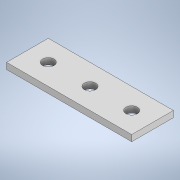
# Autodesk Inventor part: X-Axis End Pulley Holder
Saved by Autodesk Inventor 2022 (Build 260153000, 153)
## iProperties
Created: 2022-12-29
Part Number: X-Axis End Pulley Holder
Material: Generic
Document SubType Name: Modeling
Designer: Gaming
Density: 1 g/cm^3
Appearance: Default
Author: Gaming
Autodesk Inventor part; units mm, degrees
ref_plane "YZ Plane" through (0, 0, 0) normal (1, 0, 0) x (0, 1, 0)
ref_plane "XZ Plane" through (0, 0, 0) normal (0, 1, 0) x (-1, 0, 0)
ref_plane "XY Plane" through (0, 0, 0) normal (0, 0, 1) x (1, 0, 0)
sketch "Sketch1" plane through (0, 0, 0) normal (0, 1, 0) x (-1, 0, 0)
  line L0 (30, 10) -> (-30, 10)
  line L1 (-30, 10) -> (-30, -10)
  line L2 (-30, -10) -> (30, -10)
  line L3 (30, -10) -> (30, 10)
  point P0 (0, 0)
  point P1 (30, 0)
  point P2 (0, -10)
  dimension "d0" = 60
  dimension "d1" = 20
  constraints: 8 end point, 2 midpoint, 2 parallel, 1 horizontal, 1 horizontal alignment, 1 perpendicular, 1 vertical alignment
  measures "d0" distance of L2.end L1.end
  measures "d1" distance of L1.end L0.end
extrude "Extrusion1" add sketch "Sketch1" along normal blind 3
sketch "Sketch2" plane through (0, 3, 0) normal (0, 1, 0) x (1, 0, 0)
  point P0 (0, 0)
  point P1 (0, 0)
  point P2 (-20, 0)
  point P3 (20, 0)
  dimension "d4" = 20
  dimension "d5" = 20
  constraints: 2 coincident, 2 horizontal alignment
  measures "d4" distance of point (-20, 0) point (0, 0)
  measures "d5" distance of point (0, 0) point (20, 0)
hole "Hole1" at (0, 3, 0) at (-20, 3, 0) at (20, 3, 0) direction (0, -1, 0) diameter 5.5 end through all
equation "\"d5\" = d4"
body "Solid1"
